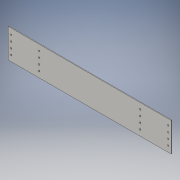
# Autodesk Inventor part: End Plates
Saved by Autodesk Inventor 2016 (Build 200138000, 138)
## iProperties
Created: 2018-05-05
Part Number: End Plates
Material: Generic
Document SubType Name: Modeling
Designer: Kade
Density: 1 g/cm^3
Appearance: Default
Sheet Metal Rule: Default
Mass: 285.073 g
Surface Area: 1859.38 cm^2
Volume: 285.073 cm^3
Author: Kade
Autodesk Inventor part; units mm, degrees
ref_plane "YZ Plane" through (0, 0, 0) normal (1, 0, 0) x (0, 1, 0)
ref_plane "XZ Plane" through (0, 0, 0) normal (0, 1, 0) x (-1, 0, 0)
ref_plane "XY Plane" through (0, 0, 0) normal (0, 0, 1) x (1, 0, 0)
sketch "Sketch3" plane through (0, 0, 0) normal (0, 0, 1) x (1, 0, 0)
  line L0 (-355.6, -63.5) -> (355.6, -63.5)
  line L1 (355.6, -63.5) -> (355.6, 63.5)
  line L2 (355.6, 63.5) -> (-355.6, 63.5)
  line L3 (-355.6, 63.5) -> (-355.6, -63.5)
  line L4 (-355.6, -63.5) -> (355.6, 63.5) construction
  line L5 (355.6, -63.5) -> (-355.6, 63.5) construction
  circle A0 centre (-342.9, 38.1) radius 3.2639
  circle A1 centre (-342.9, 12.7) radius 3.2639
  circle A2 centre (-342.9, -12.7) radius 3.2639
  circle A3 centre (-342.9, -38.1) radius 3.2639
  line L6 (-233.6038, 63.5) -> (-233.6038, -63.5)
  circle A4 centre (-220.9038, 38.1) radius 3.2639
  circle A5 centre (-220.9038, 12.7) radius 3.2639
  circle A6 centre (-220.9038, -12.7) radius 3.2639
  circle A7 centre (-220.9038, -38.1) radius 3.2639
  line L7 (0, 63.5) -> (0, -63.5) construction
  circle A8 centre (342.9, 38.1) radius 3.2639
  circle A9 centre (342.9, 12.7) radius 3.2639
  circle A10 centre (342.9, -12.7) radius 3.2639
  circle A11 centre (342.9, -38.1) radius 3.2639
  circle A12 centre (220.9038, 38.1) radius 3.2639
  circle A13 centre (220.9038, 12.7) radius 3.2639
  circle A14 centre (220.9038, -12.7) radius 3.2639
  circle A15 centre (220.9038, -38.1) radius 3.2639
  point P0 (0, 0)
  dimension "d58" = 711.2
  dimension "d59" = 127
  dimension "d60" = 6.5278
  dimension "d61" = 6.5278
  dimension "d62" = 6.5278
  dimension "d63" = 6.5278
  dimension "d64" = 25.4
  dimension "d65" = 25.4
  dimension "d66" = 25.4
  dimension "d69" = 0
  dimension "d70" = 0
  dimension "d71" = 0
  dimension "d72" = 25.4
  dimension "d73" = 25.4
  dimension "d74" = 12.7
  dimension "d77" = 121.9962
  dimension "d82" = 127
  constraints: 16 centre point, 16 end point, 8 symmetric about line, 4 midpoint, 2 horizontal, 2 parallel, 1 perpendicular, 19 other
  measures "d58" distance of L0.start L0.end
  measures "d59" distance of L1.end L0.end
  measures "d60" diameter of A0
  measures "d61" diameter of A1
  measures "d62" diameter of A2
  measures "d63" diameter of A3
  measures "d64" distance of A2.centre A3.centre
  measures "d65" distance of A1.centre A2.centre
  measures "d66" distance of A0.centre A1.centre
  measures "d69" horizontal distance of A2.centre A3.centre
  measures "d70" horizontal distance of A1.centre A2.centre
  measures "d71" horizontal distance of A0.centre A1.centre
  measures "d72" distance from line of L0 A3.centre
  measures "d73" distance from line of A0.centre L2
  measures "d74" distance from line of L3 A0.centre
  measures "d77" distance of L2.end L6.start
  measures "d82" distance of L7.start L7.end
extrude "Extrusion3" add sketch "Sketch3" along normal blind 3.175
equation "\"d72\" = d73"
equation "\"BendRadius\" = Thickness"
equation "\"BendReliefWidth\" = Thickness"
equation "\"BendReliefDepth\" = 0.5 * Thickness"
equation "\"CornerReliefSize\" = 4 * Thickness"
equation "\"MinimumRemnant\" = 2 * Thickness"
equation "\"TransitionRadius\" = BendRadius"
equation "\"JacobiRadiusSize\" = Thickness"
equation "\"GapSize\" = Thickness"
equation "\"Thickness\" = 3.048"
body "Solid2"
